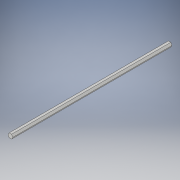
# Autodesk Inventor part: Hex Shaft ARm
Saved by Autodesk Inventor 2018 (Build 220112000, 112)
## iProperties
Created: 2019-01-23
Part Number: Hex Shaft ARm
Material: Generic
Document SubType Name: Modeling
Designer: Gabriel
Density: 1 g/cm^3
Appearance: Default
Author: Gabriel
Autodesk Inventor part; units mm, degrees
ref_plane "YZ Plane" through (0, 0, 0) normal (1, 0, 0) x (0, 1, 0)
ref_plane "XZ Plane" through (0, 0, 0) normal (0, 1, 0) x (-1, 0, 0)
ref_plane "XY Plane" through (0, 0, 0) normal (0, 0, 1) x (1, 0, 0)
sketch "Sketch1" plane through (0, 0, 0) normal (0, 0, 1) x (1, 0, 0)
  line L0 (0, 0) -> (0, 6.35) construction
  line L1 (3.6591, 6.35) -> (7.3288, 0.0061)
  line L2 (7.3288, 0.0061) -> (3.6697, -6.3439)
  line L3 (3.6697, -6.3439) -> (-3.6591, -6.35)
  line L4 (-3.6591, -6.35) -> (-7.3288, -0.0061)
  line L5 (-7.3288, -0.0061) -> (-3.6697, 6.3439)
  line L6 (-3.6697, 6.3439) -> (3.6591, 6.35)
  dimension "d0" = 6.35
  constraints: 14 end point, 1 coincident, 1 vertical, 13 other
  measures "d0" distance of L0.start L0.end
extrude "Extrusion1" add sketch "Sketch1" along normal blind 482.6
body "Solid1"
